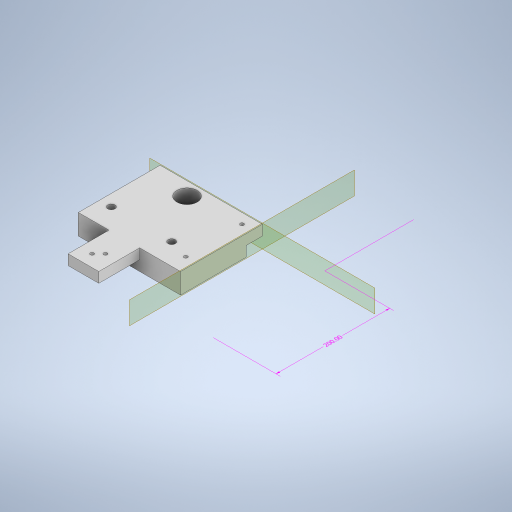
# Autodesk Inventor part: base_mid_3
Saved by Autodesk Inventor 2023 (Build 270158000, 158)
## iProperties
Created: 2022-11-29
Part Number: base_mid_3
Material: Genérico
Document SubType Name: Modeling
Designer: inigo
Density: 1 g/cm^3
Appearance: Valor por defecto
Author: inigo
Autodesk Inventor part; units mm, degrees
ref_plane "YZ Plane" through (0, 0, 0) normal (1, 0, 0) x (0, 1, 0)
ref_plane "XZ Plane" through (0, 0, 0) normal (0, 1, 0) x (-1, 0, 0)
ref_plane "XY Plane" through (0, 0, 0) normal (0, 0, 1) x (1, 0, 0)
sketch "Boceto1" plane through (0, 0, 0) normal (0, 1, 0) x (-1, 0, 0)
  line L0 (100, 80) -> (-100, 80)
  line L1 (-100, 80) -> (-100, -80)
  line L2 (-100, -80) -> (100, -80)
  line L3 (100, -80) -> (100, 80)
  line L4 (100, 80) -> (-100, -80) construction
  line L5 (-100, 80) -> (100, -80) construction
  point P0 (0, 0)
  dimension "d0" = 200
  dimension "d1" = 160
  constraints: 12 end point, 2 midpoint, 2 parallel, 1 horizontal, 1 perpendicular
  measures "d0" distance of L2.end L1.end
  measures "d1" distance of L1.end L0.end
extrude "Extrusión1" add sketch "Boceto1" along normal blind 20
sketch "Boceto2" plane through (0, 20, 0) normal (0, 1, 0) x (1, 0, 0)
  line L0 (-100, 80) -> (-100, -80) projected
  line L1 (-100, 80) -> (-70, 80)
  line L2 (-70, 80) -> (-70, 40)
  line L3 (-70, 40) -> (-100, 40)
  line L4 (-100, 40) -> (-100, 80)
  line L5 (100, 80) -> (-100, 80) projected
  line L6 (0, 80) -> (0, 40)
  line L7 (100, 80) -> (70, 80)
  line L8 (70, 80) -> (70, 40)
  line L9 (70, 40) -> (100, 40)
  line L10 (100, 40) -> (100, 80)
  point P0 (0, 0)
  dimension "d4" = 30
  dimension "d5" = 40
  constraints: 18 end point, 3 symmetric about line, 2 parallel, 1 horizontal, 1 midpoint, 1 perpendicular, 1 vertical
  measures "d4" distance of L2.end L3.end
  measures "d5" distance of L1.end L2.end
extrude "Extrusión2" cut sketch "Boceto2" against normal blind 10
sketch "Boceto3" plane through (0, 20, 0) normal (0, 1, 0) x (1, 0, 0)
  line L0 (-70, 80) -> (-70, 40) projected
  line L1 (-70, 80.0001) -> (-70, 40)
  line L2 (-70, 40) -> (-100, 40) projected
  line L3 (-100, 40) -> (-100, 80.0001)
  line L4 (-100, 40) -> (-70, 40)
  line L5 (-70, 40) -> (-70, 80)
  line L6 (-70, 80) -> (-100, 80)
  line L7 (-100, 80) -> (-100, 40)
  circle A0 centre (-88.25, 58.25) radius 1.75
  circle A1 centre (-81.75, 51.75) radius 1.75
  line L8 (100, 80) -> (-100, 80) projected
  line L9 (0, 80) -> (0, 56.5)
  circle A2 centre (88.25, 58.25) radius 1.75
  circle A3 centre (81.75, 51.75) radius 1.75
  point P0 (0, 0)
  point P1 (-64.3507, 80)
  point P2 (-74.3507, 0)
  point P3 (-85, 80)
  dimension "d23" = 21.75
  dimension "d24" = 11.75
  dimension "d26" = 11.75
  constraints: 14 end point, 4 centre point, 3 vertical, 2 midpoint, 2 parallel, 2 symmetric about line, 1 horizontal, 1 perpendicular, 2 other
  measures "d23" vertical distance of point (-85, 80) A0.centre
  measures "d24" distance from line of L3 A0.centre
  measures "d26" distance from line of L0 A1.centre
hole "Agujero1" at (-81.75, 20, -51.75) at (-88.25, 20, -58.25) at (81.75, 20, -51.75) at (88.25, 20, -58.25) direction (0, -1, 0) diameter 3.5 end through all
sketch "Boceto4" plane through (-100, 0, 80) normal (0, 0, 1) x (1, 0, 0)
  line L0 (30, 20) -> (60, 20)
  line L1 (60, 20) -> (60, 10)
  line L2 (60, 10) -> (30, 10)
  line L3 (30, 10) -> (30, 20)
  line L4 (0, 0) -> (0, 20) projected
  line L5 (100, 0) -> (100, 10)
  line L6 (170, 20) -> (140, 20)
  line L7 (140, 20) -> (140, 10)
  line L8 (140, 10) -> (170, 10)
  line L9 (170, 10) -> (170, 20)
  dimension "d34" = 30
  dimension "d35" = 10
  dimension "d36" = 30
  constraints: 18 end point, 4 symmetric about line, 2 parallel, 1 horizontal, 1 perpendicular, 1 vertical
  measures "d34" distance of L1.end L2.end
  measures "d35" distance of L0.end L1.end
  measures "d36" distance between parallel lines of L4 L3
extrude "Extrusión3" add sketch "Boceto4" along normal blind 40
sketch "Boceto5" plane through (0, 20, 0) normal (0, 1, 0) x (1, 0, 0)
  line L0 (59.9999, -50) -> (69.9999, -50)
  line L1 (49.9999, -101.75) -> (49.9999, -79.9497)
  line L2 (59.9999, -108.25) -> (59.9999, -50)
  line L3 (40, -80) -> (69.9999, -80)
  line L4 (49.9999, -79.9497) -> (40, -80)
  circle A0 centre (51.7499, -101.75) radius 1.75
  circle A1 centre (58.2499, -108.25) radius 1.75
  line L5 (69.9999, -80) -> (69.9999, -120)
  line L6 (40, -120) -> (40, -80)
  line L7 (69.9999, -120) -> (40, -120)
  line L8 (0, -50) -> (0, -71.75)
  line L9 (-40, -120) -> (-40, -80)
  line L10 (-49.9999, -101.75) -> (-49.9999, -79.9497)
  circle A2 centre (-51.7499, -101.75) radius 1.75
  circle A3 centre (-58.2499, -108.25) radius 1.75
  line L11 (-40, -80) -> (-69.9999, -80)
  line L12 (-69.9999, -120) -> (-40, -120)
  line L13 (-69.9999, -80) -> (-69.9999, -120)
  line L14 (-59.9999, -108.25) -> (-59.9999, -50)
  line L15 (-40, -120) -> (-69.9999, -120)
  line L16 (-69.9999, -80) -> (-69.9999, -120)
  line L17 (-40, -120) -> (-70, -120) projected
  line L18 (-40, -80) -> (-40, -120) projected
  line L19 (-59.9999, -110) -> (-49.9999, -110)
  line L20 (-49.9999, -110) -> (-49.9999, -100)
  line L21 (-49.9999, -100) -> (-59.9999, -100)
  line L22 (-59.9999, -100) -> (-59.9999, -110)
  line L23 (-100, 40) -> (-100, -80) projected
  point P0 (0, 0)
  point P1 (-56.75, -68.25)
  point P2 (-63.25, -61.75)
  point P3 (63.25, -61.75)
  point P4 (56.75, -68.25)
  dimension "d45" = 3.5
  dimension "d46" = 3.5
  dimension "d39" = 10
  dimension "d40" = 10
  dimension "d41" = 40
  dimension "d42" = 0
  dimension "d43" = 6.5
  dimension "d44" = 6.5
  dimension "d47" = 11.7499
  dimension "d48" = 11.75
  dimension "d49" = 0
  dimension "d50" = 11.75
  dimension "d51" = 0
  dimension "d97" = 40.0001
  constraints: 42 end point, 10 symmetric about line, 6 vertical, 4 horizontal alignment, 4 parallel, 2 horizontal, 2 perpendicular, 1 point on line, 8 other
  measures "d39" distance of L1.end L3.start
  measures "d40" distance of L0.start L0.end
  measures "d41" distance of L3.end L5.end
  measures "d42" distance between parallel lines of L15 L12
  measures "d43" horizontal distance of point (-58.25, -108.25) point (-51.75, -101.75)
  measures "d44" horizontal distance of point (-58.25, -108.25) point (-51.75, -101.75)
  measures "d47" distance from line of L9 point (-51.75, -101.75)
  measures "d48" distance from line of L13 point (-58.25, -108.25)
  measures "d49" distance between parallel lines of L17 L12
  measures "d50" distance from line of L12 point (-58.25, -108.25)
  measures "d51" distance between parallel lines of L18 L9
  measures "d97" distance between parallel lines of L23 L22
hole "Agujero2" at (-58.2499, 20, 108.25) at (-51.7499, 20, 101.75) at (51.7499, 20, 101.75) at (58.2499, 20, 108.25) direction (0, -1, 0) diameter 3.5 end through all
sketch "Boceto6" plane through (0, 20, 0) normal (0, 1, 0) x (1, 0, 0)
  circle A0 centre (-60.569, -13.1067) radius 10
  circle A1 centre (-29.569, -59.1067) radius 3.5
  line L0 (-60.569, -13.1067) -> (-39.0083, -13.1067)
  circle A2 centre (-29.569, 25.8933) radius 3.5
  circle A3 centre (-88.569, 25.8933) radius 3.5
  circle A4 centre (-88.569, -59.1067) radius 3.5
  line L1 (70.4544, -63.0517) -> (18.4544, -63.0517)
  line L2 (18.4544, -63.0517) -> (18.4544, 6.9483)
  line L3 (18.4544, 6.9483) -> (70.4544, 6.9483)
  line L4 (70.4544, 6.9483) -> (70.4544, -63.0517)
  line L5 (70.4544, 6.9483) -> (48.4544, 6.9483)
  line L6 (48.4544, 6.9483) -> (48.4544, 48.9483)
  line L7 (48.4544, 48.9483) -> (70.4544, 48.9483)
  line L8 (70.4544, 48.9483) -> (70.4544, 6.9483)
  line L9 (77.2288, -8.158) -> (77.2281, -5.6604)
  circle A5 centre (63.7706, -5.7606) radius 1.75
  line L10 (70.7641, -24.1464) -> (70.7641, 22.2796)
  circle A6 centre (35.8307, -5.7609) radius 1.75
  line L11 (25.1581, -13.2381) -> (25.1581, -10.7404)
  circle A7 centre (68.8507, -57.8309) radius 1.75
  line L12 (26.4277, 35.0051) -> (26.4277, 37.5029)
  circle A8 centre (20.6074, -56.5614) radius 1.75
  line L13 (18.6941, -55.9176) -> (70.7641, -55.9176)
  line L14 (18.6941, -55.9176) -> (18.6941, -7.6743)
  line L15 (44.7291, -55.9176) -> (44.7291, -31.7959)
  line L16 (63.7706, -28.0517) -> (26.4277, -28.0517)
  line L17 (44.7291, -23.5247) -> (44.7291, -31.7959)
  point P0 (0, 0)
  point P1 (-60.569, -16.6067)
  point P2 (45.425, 12.8886)
  point P3 (44.7291, -28.0517)
  dimension "d59" = 7
  dimension "d60" = 7
  dimension "d61" = 7
  dimension "d62" = 39
  dimension "d63" = 46
  dimension "d64" = 59
  dimension "d65" = 46
  dimension "d66" = 39
  dimension "d67" = 59
  dimension "d68" = 52
  dimension "d69" = 70
  dimension "d70" = 22
  dimension "d71" = 42
  dimension "d72" = 3.5
  dimension "d73" = 3.5
  dimension "d74" = 3.5
  dimension "d75" = 3.5
  dimension "d142" = 17.3763
  dimension "d143" = 12.7092
  dimension "d144" = 6.6837
  dimension "d145" = 12.7089
  dimension "d146" = 5.2208
  dimension "d147" = 1.6037
  dimension "d148" = 2.1531
  dimension "d149" = 6.4903
  constraints: 36 end point, 9 centre point, 5 parallel, 3 perpendicular, 2 point on line, 1 horizontal, 1 midpoint
  measures "d59" diameter of A1
  measures "d60" diameter of A2
  measures "d61" diameter of A4
  measures "d62" vertical distance of L0.start A3.centre
  measures "d63" vertical distance of L0.start A4.centre
  measures "d64" distance of A4.centre A1.centre
  measures "d65" vertical distance of L0.start A1.centre
  measures "d66" vertical distance of A2.centre L0.start
  measures "d67" distance between centres of A3 A2
  measures "d68" distance of L2.end L3.end
  measures "d69" distance of L1.end L2.end
  measures "d70" distance of L6.end L7.end
  measures "d71" distance of L5.end L6.end
  measures "d72" diameter of A5
  measures "d73" diameter of A6
  measures "d74" diameter of A7
  measures "d75" diameter of A8
  measures "d142" distance from line of L2 A6.centre
  measures "d143" distance from line of L3 A6.centre
  measures "d144" distance from line of L4 A5.centre
  measures "d145" distance from line of L3 A5.centre
  measures "d146" distance from line of L1 A7.centre
  measures "d147" distance from line of L4 A7.centre
  measures "d148" distance from line of L2 A8.centre
  measures "d149" distance from line of L1 A8.centre
hole "Agujero3" at (68.8507, 20, 57.8309) at (20.6074, 20, 56.5614) at (63.7706, 20, 5.7606) at (35.8307, 20, 5.7609) direction (0, -1, 0) diameter 3.5 end through all
sketch "Boceto7" plane through (0, 20, 0) normal (0, 1, 0) x (1, 0, 0)
  circle A0 centre (-60.569, -13.1067) radius 10
  circle A1 centre (-29.569, -59.1067) radius 3.5
  line L0 (-60.569, -13.1067) -> (-39.0083, -13.1067)
  circle A2 centre (-29.569, 25.8933) radius 3.5
  circle A3 centre (-88.569, 25.8933) radius 3.5
  circle A4 centre (-88.569, -59.1067) radius 3.5
  point P0 (0, 0)
  point P1 (-60.569, -16.6067)
  dimension "d83" = 7
  dimension "d84" = 7
  dimension "d85" = 7
  dimension "d86" = 39
  dimension "d87" = 46
  dimension "d88" = 59
  dimension "d89" = 46
  dimension "d90" = 39
  dimension "d91" = 59
  constraints: 5 centre point, 2 end point, 1 horizontal
  measures "d83" diameter of A1
  measures "d84" diameter of A2
  measures "d85" diameter of A4
  measures "d86" vertical distance of L0.start A3.centre
  measures "d87" vertical distance of L0.start A4.centre
  measures "d88" distance of A4.centre A1.centre
  measures "d89" vertical distance of L0.start A1.centre
  measures "d90" vertical distance of A2.centre L0.start
  measures "d91" distance between centres of A3 A2
extrude "Extrusión4" cut sketch "Boceto7" against normal blind 20
ref_plane "Plano de trabajo1" through (0, 0, -80) normal (-1, 0, 0) x (0, 0, 1)
ref_plane "Plano de trabajo2" through (100, 0, 0) normal (0, 0, -1) x (-1, 0, 0)
sketch "Boceto8" plane through (0, 20, 0) normal (0, 1, 0) x (1, 0, 0)
  line L0 (80, -15) -> (90, -15)
  circle A0 centre (85, -10) radius 1.75
  line L1 (85, 10) -> (85, -10)
  line L2 (90, -15) -> (90, 15)
  circle A1 centre (85, 10) radius 1.75
  line L3 (80, 15) -> (80, -15)
  line L4 (90, 15) -> (80, -15) construction
  line L5 (80, 15) -> (90, -15) construction
  line L6 (90, 15) -> (80, 15)
  line L7 (100, -80) -> (100, 40) projected
  line L8 (0, 0) -> (20, -20)
  line L9 (0, 0) -> (28.2843, 0) construction
  line L10 (15, -60) -> (15, -70)
  circle A2 centre (10, -65) radius 1.75
  line L11 (-10, -65) -> (10, -65)
  line L12 (15, -70) -> (-15, -70)
  circle A3 centre (-10, -65) radius 1.75
  line L13 (-15, -60) -> (15, -60)
  line L14 (-15, -70) -> (15, -60) construction
  line L15 (-15, -60) -> (15, -70) construction
  line L16 (-15, -70) -> (-15, -60)
  line L17 (0, 0) -> (18.6615, 18.6615)
  line L18 (0, 0) -> (26.3913, 0) construction
  line L19 (-15, 60) -> (-15, 70)
  circle A4 centre (-10, 65) radius 1.75
  line L20 (10, 65) -> (-10, 65)
  line L21 (-15, 70) -> (15, 70)
  circle A5 centre (10, 65) radius 1.75
  line L22 (15, 60) -> (-15, 60)
  line L23 (15, 70) -> (-15, 60) construction
  line L24 (15, 60) -> (-15, 70) construction
  line L25 (15, 70) -> (15, 60)
  line L26 (70, 80) -> (-70, 80) projected
  line L27 (-40, -80) -> (40, -80) projected
  point P0 (86.9608, 0)
  point P1 (86.9608, 0)
  point P2 (85, 15)
  point P3 (0, -69.1269)
  point P4 (0, -69.1269)
  point P5 (-15, -67.1661)
  point P6 (0, 69.7066)
  point P7 (0, 69.7066)
  point P8 (15, 67.7458)
  point P9 (-15, 65)
  point P10 (15, -65)
  dimension "d98" = 10
  dimension "d99" = 30
  dimension "d100" = 10
  dimension "d101" = 5
  dimension "d102" = 5
  dimension "d103" = 5
  dimension "d104" = 5
  dimension "d105" = 45
  dimension "d106" = 45
  dimension "d107" = 10
  dimension "d108" = 10
  dimension "d109" = 30
  dimension "d110" = 5
  dimension "d111" = 5
  dimension "d112" = 5
  dimension "d113" = 5
  dimension "d114" = 10
  dimension "d115" = 30
  dimension "d116" = 5
  dimension "d117" = 5
  dimension "d118" = 5
  dimension "d119" = 5
  dimension "d120" = 10
  constraints: 32 end point, 6 centre point, 3 midpoint, 2 equal length, 2 horizontal, 27 other
  measures "d98" distance between parallel lines of L2 L7
  measures "d99" distance between parallel lines of L0 L6
  measures "d100" distance between parallel lines of L2 L3
  measures "d101" distance from line of L2 A0.centre
  measures "d102" distance from line of L0 A0.centre
  measures "d103" distance from line of L2 A1.centre
  measures "d104" distance of point (85, 15) A1.centre
  measures "d105" angle of L8 L9
  measures "d106" angle of L18 L17
  measures "d107" distance between parallel lines of L21 L26
  measures "d108" distance between parallel lines of L22 L21
  measures "d109" distance between parallel lines of L25 L19
  measures "d110" distance from line of L25 A5.centre
  measures "d111" distance from line of L21 A5.centre
  measures "d112" distance from line of L21 A4.centre
  measures "d113" distance of point (-15, 65) A4.centre
  measures "d114" distance between parallel lines of L12 L13
  measures "d115" distance between parallel lines of L16 L10
  measures "d116" distance of point (15, -65) A2.centre
  measures "d117" distance from line of L13 A2.centre
  measures "d118" distance from line of L13 A3.centre
  measures "d119" distance from line of L16 A3.centre
  measures "d120" distance between parallel lines of L27 L12
hole "Agujero4" at (-10, 20, -65) at (10, 20, -65) at (85, 20, -10) at (85, 20, 10) at (10, 20, 65) at (-10, 20, 65) direction (0, -1, 0) diameter 3.5 end through all
sketch "Boceto9" plane through (0, 20, 0) normal (0, 1, 0) x (1, 0, 0)
  circle A0 centre (10, -10) radius 1.75
  line L0 (6.803, 0) -> (14.6069, 0)
  line L1 (0, 0) -> (0, -4.8284)
  line L2 (0, 0) -> (20.0354, 0)
  circle A1 centre (10, 10) radius 1.75
  line L3 (0, 0) -> (0, 4.8284)
  circle A2 centre (-10, 10) radius 1.75
  circle A3 centre (-10, -10) radius 1.75
  dimension "d128" = 3.5
  dimension "d129" = 10
  dimension "d130" = 10
  constraints: 8 end point, 4 centre point, 4 symmetric about line, 2 horizontal, 1 vertical, 3 other
  measures "d128" diameter of A0
  measures "d129" distance from line of L1 A0.centre
  measures "d130" distance from line of L2 A0.centre
hole "Agujero5" at (-10, 20, 10) at (-10, 20, -10) at (10, 20, -10) at (10, 20, 10) direction (0, -1, 0) diameter 3.5 end through all
sketch "Boceto10" plane through (0, 0, 0) normal (0, -1, 0) x (1, 0, 0)
  line L0 (-16, 16) -> (16, 16)
  line L1 (16, 16) -> (16, -16)
  line L2 (16, -16) -> (-16, -16)
  line L3 (-16, -16) -> (-16, 16)
  line L4 (-16, 16) -> (16, -16) construction
  line L5 (16, 16) -> (-16, -16) construction
  point P0 (0, 0)
  point P1 (0, 0)
  dimension "d138" = 32
  dimension "d139" = 32
  constraints: 12 end point, 2 midpoint, 2 parallel, 1 horizontal, 1 perpendicular
  measures "d138" distance of L1.end L2.end
  measures "d139" distance of L0.end L1.end
extrude "Extrusión5" cut sketch "Boceto10" against normal blind 10
split "Dividir1" plane through (100, 0, 0) removes the side toward (0, 0, -1)
split "Dividir2" plane through (0, 0, -80) removes the side toward (1, 0, 0)
